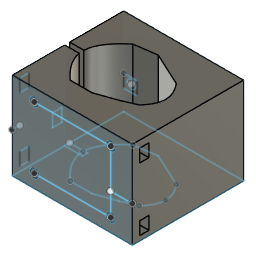
pipette_mount_i2 (Autodesk Fusion 360 design; units mm, degrees)
part number: 2026-04-21-03-05-20-879
Autodesk Fusion 360 part; units mm, degrees
sketch "Sketch1" plane through (0, 0, 0) normal (0, 0, 1) x (1, 0, 0)
  line L0 (-21.8, 22.2397) -> (26.7, 22.2397)
  line L1 (26.7, 22.2397) -> (26.7, -22.7603)
  line L2 (26.7, -22.7603) -> (-21.8, -22.7603)
  line L3 (-21.8, -22.7603) -> (-21.8, 22.2397)
  spline S0 degree 5 poles (-8.2949, 12.4487) (-8.8839, 11.9576) (-10.0102, 10.9741) (-11.5448, 9.495) (-13.2761, 7.5148) (-14.8799, 5.0253) (-15.8741, 2.5205) (-16.2099, -0.001) (-15.8626, -2.5398) (-14.8614, -5.0951) (-13.2565, -7.6657) (-11.5298, -9.7334) (-10.0015, -11.2901) (-8.8808, -12.3304) (-8.2949, -12.8513) knots 0 0 0 0 0 0 0.1 0.2 0.3 0.4 0.5 0.6 0.7 0.8 0.9 1 1 1 1 1 1
  spline S1 degree 5 poles (14.2993, 7.4153) (14.5562, 7.1034) (15.0477, 6.4806) (15.718, 5.5494) (16.4756, 4.3142) (17.1805, 2.7814) (17.6209, 1.2609) (17.7748, -0.2462) (17.6287, -1.7394) (17.193, -3.2192) (16.4888, -4.6864) (15.7281, -5.8511) (15.0535, -6.7197) (14.5583, -7.2967) (14.2993, -7.5847) knots 0 0 0 0 0 0 0.1 0.2 0.3 0.4 0.5 0.6 0.7 0.8 0.9 1 1 1 1 1 1
  line L4 (-21.8, -1.6206) -> (-14.6097, -1.6206)
  line L5 (-14.6097, -1.6206) -> (-14.6097, 0.3794)
  line L6 (-14.6097, 0.3794) -> (-21.8, 0.3794)
  line L7 (14.2993, 7.4153) -> (0.6904, 13.733)
  line L8 (0.6904, 13.733) -> (-8.2949, 12.4487)
  line L9 (0.4715, -12.8513) -> (-8.2949, -12.8513)
  line L10 (14.2993, -7.5847) -> (8.5702, -10.0161)
  line L11 (8.5702, -10.0161) -> (0.4715, -12.8513)
  point P0 (-16.0393, 0.095)
  point P1 (17.6997, -0.3339)
  dimension "d6" = 48.5
  dimension "d7" = 45
  dimension "d8" = 15
  dimension "d9" = 25.3
  dimension "d11" = 2
  constraint horizontal L0
  constraint vertical L1
  constraint horizontal L2
  constraint vertical L3
  constraint horizontal L4
  constraint vertical L5
  constraint horizontal L6
  constraint coincident L3 L4.start
  constraint horizontal L9
  measures "d6" distance of L0.start L0.end
  measures "d7" distance of L0.start L2.end
  measures "d8" distance of S1.end S1.start
  measures "d9" distance of S0.end S0.start
  measures "d11" distance of L4.start L6.end
extrude "Extrude1" add sketch "Sketch1" along normal blind 35.3 contours L0 L1 L2 L3 S0 S1 L4 L6 L7 L8 L9 L10 L11
sketch "bad_sketch" plane through (0, 0, 0) normal (0, 0, 1) x (1, 0, 0)
  line L0 (24.6924, 6.1679) -> (15.4617, 8.9936)
  line L1 (15.4617, 8.9936) -> (5.166, 12.1454)
  line L2 (5.166, 12.1454) -> (-5.166, 12.8182)
  line L3 (-5.166, 12.8182) -> (-14.9618, 9.182)
  line L4 (-14.9618, 9.182) -> (-20.3307, 2.1177)
  line L5 (-20.3307, 2.1177) -> (-20.3307, -2.686)
  line L6 (-20.3307, -2.686) -> (-14.9618, -8.9968)
  line L7 (-14.9618, -8.9968) -> (-10.0639, -11.3515)
  line L8 (-10.0639, -11.3515) -> (-5.166, -12.4818)
  line L9 (-5.166, -12.4818) -> (5.166, -12.4818)
  line L10 (5.166, -12.4818) -> (10.3139, -11.0689)
  line L11 (10.3139, -11.0689) -> (24.6924, -8.2432)
  line L12 (24.6924, -8.2432) -> (28.2717, -1.8383)
  line L13 (28.2717, -1.8383) -> (28.9264, 0.3007)
  line L14 (28.9264, 0.3007) -> (26.482, 5.6201)
  line L15 (26.482, 5.6201) -> (24.6924, 6.1679)
  line L16 (-28.837, -17.65) -> (19.663, -17.65)
  line L17 (19.663, -17.65) -> (19.663, 27.35)
  line L18 (19.663, 27.35) -> (-28.837, 27.35)
  line L19 (-28.837, 27.35) -> (-28.837, -17.65)
  line L20 (-28.837, -1.4888) -> (-19.0112, -1.4888)
  line L21 (-19.0112, -1.4888) -> (-19.0112, 0.5112)
  line L22 (-19.0112, 0.5112) -> (-28.837, 0.5112)
  line L23 (-28.837, 0.5112) -> (-28.837, -1.4888)
  dimension "d15" = 48.5
  dimension "d16" = 45
  dimension "d17" = 2
  constraint parallel L0 L1
  constraint horizontal L9
  constraint perpendicular L0 L13
  constraint perpendicular L13 L15
  constraint horizontal L16
  constraint vertical L17
  constraint horizontal L18
  constraint vertical L19
  constraint horizontal L20
  constraint vertical L21
  constraint horizontal L22
  constraint vertical L23
  constraint coincident L19 L20.start
  measures "d15" distance of L16.start L16.end
  measures "d16" distance of L16.start L18.end
  measures "d17" distance of L20.start L22.end
sketch "Sketch3" plane through (0, 22.2397, 0) normal (0, 1, 0) x (-1, 0, 0)
  line L0 (-26.7, 0) -> (21.8, 0)
  line L1 (21.8, 0) -> (21.8, 35.3)
  line L2 (21.8, 35.3) -> (-26.7, 35.3)
  line L3 (-26.7, 35.3) -> (-26.7, 0)
  circle A0 centre (18.6487, 11.1813) radius 1.7
  line L4 (21.8, 13.5098) -> (16.4, 13.5098)
  line L5 (16.4, 13.5098) -> (16.4, 8.2098)
  line L6 (16.4, 8.2098) -> (21.8, 8.2098)
  line L7 (21.8, 8.2098) -> (21.8, 13.5098)
  dimension "d23" = 3.4
  dimension "d26" = 5.4
  dimension "d27" = 5.3
  constraint horizontal L4
  constraint vertical L5
  constraint horizontal L6
  constraint vertical L7
  constraint coincident L1 L4.start
  measures "d23" diameter of A0
  measures "d26" distance of L4.start L4.end
  measures "d27" distance of L4.start L6.end
hole "Hole1" at (-18.6487, 22.2397, 11.1813) direction (0, -1, 0) diameter 3.4 depth 26 tip angle 180
extrude "Extrude3" cut sketch "Sketch3" against normal blind 16 contours L1 L4 L5 L6 L7
sketch "Sketch4" plane through (0, -22.7603, 0) normal (0, -1, 0) x (1, 0, 0)
  line L0 (-21.8, 0) -> (26.7, 0)
  line L1 (26.7, 0) -> (26.7, 35.3)
  line L2 (26.7, 35.3) -> (-21.8, 35.3)
  line L3 (-21.8, 35.3) -> (-21.8, 0)
  line L4 (18.0274, 30.3462) -> (-12.9426, 30.3462)
  line L5 (18.0274, 30.3462) -> (18.0274, 5.3462)
  line L6 (18.0274, 5.3462) -> (-12.9426, 5.3462)
  circle A0 centre (18.0274, 5.3462) radius 1.6
  circle A1 centre (-12.9426, 5.3462) radius 1.6
  circle A2 centre (18.0274, 30.3462) radius 1.6
  circle A3 centre (-12.9426, 30.3462) radius 1.6
  line L7 (26.7, 14.5722) -> (17.935, 14.5722)
  dimension "d36" = 30.97
  dimension "d38" = 25
  dimension "d40" = 30.97
  dimension "d41" = 3.2
  dimension "d42" = 3.2
  dimension "d43" = 3.2
  dimension "d44" = 3.2
  dimension "d45" = 8.765
  constraint parallel L2 L4
  constraint perpendicular L4 L5
  constraint perpendicular L5 L6
  constraint coincident L5.end L6.start
  constraint coincident L6.end A1.centre
  constraint coincident L4.start L5.start
  constraint coincident L4.end A3.centre
  constraint coincident L1 L7.start
  constraint perpendicular L1 L7
  measures "d36" distance of L4.start L4.end
  measures "d38" distance of L4.start L5.end
  measures "d40" distance of L5.end L6.end
  measures "d41" diameter of A0
  measures "d42" diameter of A1
  measures "d43" diameter of A2
  measures "d44" diameter of A3
  measures "d45" distance of L7.start L7.end
hole "Hole2" at (18.0274, -22.7603, 5.3462) at (-12.9426, -22.7603, 5.3462) at (18.0274, -22.7603, 30.3462) at (-12.9426, -22.7603, 30.3462) direction (0, 1, 0) diameter 3.2 depth 12 tip angle 180
sketch "Sketch5" plane through (-21.8, 0, 0) normal (-1, 0, 0) x (0, -1, 0)
  line L0 (1.6206, 0) -> (22.7603, 0)
  line L1 (22.7603, 0) -> (22.7603, 35.3)
  line L2 (22.7603, 35.3) -> (1.6206, 35.3)
  line L3 (1.6206, 35.3) -> (1.6206, 0)
  line L4 (22.7603, 16.2062) -> (19.7603, 16.2062)
  line L5 (19.7603, 7.0647) -> (16.0603, 7.0647)
  line L6 (16.0603, 7.0647) -> (16.0603, 1.8647)
  line L7 (16.0603, 1.8647) -> (19.7603, 1.8647)
  line L8 (19.7603, 1.8647) -> (19.7603, 7.0647)
  line L9 (19.7603, 27.5787) -> (16.0603, 27.5787)
  line L10 (16.0603, 27.5787) -> (16.0603, 32.7787)
  line L11 (16.0603, 32.7787) -> (19.7603, 32.7787)
  line L12 (19.7603, 32.7787) -> (19.7603, 27.5787)
  line L13 (6.4749, 8.7948) -> (2.7749, 8.7948)
  line L14 (2.7749, 8.7948) -> (2.7749, 13.9948)
  line L15 (2.7749, 13.9948) -> (6.4749, 13.9948)
  line L16 (6.4749, 13.9948) -> (6.4749, 8.7948)
  dimension "d55" = 3
  dimension "d56" = 3.7
  dimension "d57" = 5.2
  dimension "d58" = 3.7
  dimension "d59" = 5.2
  dimension "d65" = 3.7
  dimension "d66" = 5.2
  constraint coincident L1 L4.start
  constraint perpendicular L1 L4
  constraint horizontal L5
  constraint vertical L6
  constraint horizontal L7
  constraint vertical L8
  constraint vertical L4.end L5.start
  constraint horizontal L9
  constraint vertical L10
  constraint horizontal L11
  constraint vertical L12
  constraint vertical L4.end L9.start
  constraint horizontal L13
  constraint vertical L14
  constraint horizontal L15
  constraint vertical L16
  measures "d55" distance of L4.start L4.end
  measures "d56" distance of L5.start L5.end
  measures "d57" distance of L5.start L7.end
  measures "d58" distance of L9.start L9.end
  measures "d59" distance of L9.start L11.end
  measures "d65" distance of L13.start L13.end
  measures "d66" distance of L13.start L15.end
extrude "Extrude4" cut sketch "Sketch5" against normal blind 12 contours L9 L10 L11 L12
extrude "Extrude5" cut sketch "Sketch5" against normal blind 12 contours L5 L6 L7 L8
extrude "Extrude6" cut sketch "Sketch5" against normal blind 5.4 contours L13 L14 L15 L16
sketch "Sketch7" plane through (26.7, 0, 0) normal (1, 0, 0) x (0, 1, 0)
  line L0 (-22.7603, 0) -> (22.2397, 0)
  line L1 (22.2397, 0) -> (22.2397, 35.3)
  line L2 (22.2397, 35.3) -> (-22.7603, 35.3)
  line L3 (-22.7603, 35.3) -> (-22.7603, 0)
  line L4 (-19.7634, 32.4808) -> (-16.0634, 32.4808)
  line L5 (-16.0634, 32.4808) -> (-16.0634, 27.2808)
  line L6 (-16.0634, 27.2808) -> (-19.7634, 27.2808)
  line L7 (-19.7634, 27.2808) -> (-19.7634, 32.4808)
  line L8 (-19.7359, 7.0548) -> (-16.0359, 7.0548)
  line L9 (-16.0359, 7.0548) -> (-16.0359, 1.8548)
  line L10 (-16.0359, 1.8548) -> (-19.7359, 1.8548)
  line L11 (-19.7359, 1.8548) -> (-19.7359, 7.0548)
  dimension "d76" = 3.7
  dimension "d77" = 5.2
  dimension "d78" = 3.7
  dimension "d79" = 5.2
  constraint horizontal L4
  constraint vertical L5
  constraint horizontal L6
  constraint vertical L7
  constraint horizontal L8
  constraint vertical L9
  constraint horizontal L10
  constraint vertical L11
  measures "d76" distance of L4.start L4.end
  measures "d77" distance of L4.start L6.end
  measures "d78" distance of L8.start L8.end
  measures "d79" distance of L8.start L10.end
extrude "Extrude8" cut sketch "Sketch7" against normal blind 12 contours L4 L5 L6 L7 | L8 L9 L10 L11
equation "syringe_height = 25.3 mm"
equation "syringe_width = 33.6 mm"
equation "height = 45 mm"
equation "width = 48.5 mm"
equation "width4 = 15 mm"
equation "d6 = width"
equation "d7 = height"
equation "d8 = width4"
equation "d9 = syringe_height"
equation "gap_width = 2 mm"
equation "d11 = gap_width"
equation "d12 = holder_depth"
equation "d15 = width"
equation "d16 = height"
equation "d17 = gap_width"
equation "length = 3 mm"
equation "holder_depth = 35.3 mm"
equation "m3_screw_diameter = 3.4 mm"
equation "d23 = m3_screw_diameter"
equation "rect_clearing_width = 5.3 mm"
equation "rect_clearing_length = 5.4 mm"
equation "d26 = rect_clearing_length"
equation "d27 = rect_clearing_width"
equation "d28 = joining_m3_screw_length"
equation "d29 = m3_screw_diameter"
equation "joining_m3_screw_length = 26 mm"
equation "d32 = -rect_clearing_distance"
equation "rect_clearing_distance = 16 mm"
equation "m3_screw_lateral_dis = 30.97 mm"
equation "d36 = m3_screw_lateral_dis"
equation "m3_screw_vertical_dis = 25 mm"
equation "d38 = m3_screw_vertical_dis"
equation "m3_diameter = 3.2 mm"
equation "d40 = m3_screw_lateral_dis"
equation "d41 = m3_diameter"
equation "d42 = m3_diameter"
equation "d43 = m3_diameter"
equation "d44 = m3_diameter"
equation "d46 = m3_screw_depth"
equation "d47 = m3_diameter"
equation "m3_screw_depth = 12 mm"
equation "nut_insert_width = 3.7 mm"
equation "nut_insert_height = 5.2 mm"
equation "screw_nut_distance = 3 mm"
equation "d55 = screw_nut_distance"
equation "d56 = nut_insert_width"
equation "d57 = nut_insert_height"
equation "d58 = nut_insert_width"
equation "d59 = nut_insert_height"
equation "d60 = -m3_screw_depth"
equation "d62 = -m3_screw_depth"
equation "d65 = nut_insert_width"
equation "d66 = nut_insert_height"
equation "d67 = -clamp_nut_depth"
equation "clamp_nut_depth = 5.4 mm"
equation "d76 = nut_insert_width"
equation "d77 = nut_insert_height"
equation "d78 = nut_insert_width"
equation "d79 = nut_insert_height"
equation "d80 = -m3_screw_depth"
